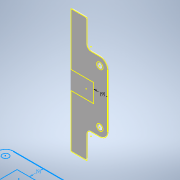
# Autodesk Inventor part: sensor_board
Saved by Autodesk Inventor 2022 (Build 260153000, 153)
## iProperties
Created: 2025-01-11
Part Number: sensor_board
Material: Типовые
Document SubType Name: Modeling
Designer: akap
Density: 1 g/cm^3
Appearance: По умолчанию
Author: akap
Autodesk Inventor part; units mm, degrees
ref_plane "YZ Plane" through (0, 0, 0) normal (1, 0, 0) x (0, 1, 0)
ref_plane "XZ Plane" through (0, 0, 0) normal (0, 1, 0) x (-1, 0, 0)
ref_plane "XY Plane" through (0, 0, 0) normal (0, 0, 1) x (1, 0, 0)
sketch "Эскиз1" plane through (0, 0, 0) normal (0, 0, 1) x (1, 0, 0)
  line L0 (0.35, -40.5) -> (-10.0814, -40.5) projected
  line L1 (0.35, -25.5) -> (0.35, -40.5) projected
  arc A0 (3.05, -22.8) -> (0.35, -25.5) centre (3.05, -25.5) ccw projected
  line L2 (8.75, -22.8) -> (3.05, -22.8) projected
  arc A1 (8.75, -22.8) -> (14.05, -17.5) centre (8.75, -17.5) ccw projected
  line L3 (14.05, 17.5) -> (14.05, -17.5) projected
  arc A2 (14.05, 17.5) -> (8.75, 22.8) centre (8.75, 17.5) ccw projected
  line L4 (3.05, 22.8) -> (8.75, 22.8) projected
  arc A3 (0.35, 25.5) -> (3.05, 22.8) centre (3.05, 25.5) ccw projected
  line L5 (0.35, 40.5) -> (0.35, 25.5) projected
  line L6 (-10.0814, 40.5) -> (0.35, 40.5) projected
  circle A4 centre (8.75, -17.5) radius 2.1 projected
  circle A5 centre (8.75, 17.5) radius 2.1 projected
  line L7 (0.05, -40.2) -> (-10.2488, -40.2)
  line L8 (-10.2488, -40.2) -> (-10.2488, 40.2)
  line L9 (-10.2488, 40.2) -> (0.05, 40.2)
  line L10 (0.05, 40.2) -> (0.05, 25.5)
  arc A6 (0.05, 25.5) -> (3.05, 22.5) centre (3.05, 25.5) ccw
  line L11 (3.05, 22.5) -> (8.75, 22.5)
  arc A7 (13.75, 17.5) -> (8.75, 22.5) centre (8.75, 17.5) ccw
  line L12 (13.75, 17.5) -> (13.75, -17.5)
  arc A8 (8.75, -22.5) -> (13.75, -17.5) centre (8.75, -17.5) ccw
  line L13 (8.75, -22.5) -> (3.05, -22.5)
  arc A9 (3.05, -22.5) -> (0.05, -25.5) centre (3.05, -25.5) ccw
  line L14 (0.05, -25.5) -> (0.05, -40.2)
  circle A10 centre (8.75, -17.5) radius 1.6
  circle A11 centre (8.75, 17.5) radius 1.6
  line L15 (-10.0814, -40.5) -> (-10.0814, -6) projected
  line L16 (-10.0814, 6) -> (-10.0814, 40.5) projected
  line L17 (-10.0814, 6) -> (4.75, 6) projected
  line L18 (4.75, 6) -> (4.75, -6) projected
  line L19 (4.75, -6) -> (-10.0814, -6) projected
  dimension "d7" = 0.3
  dimension "d8" = 3.2
  dimension "d9" = 3.2
  constraints: 16 end point, 8 point on circle, 6 centre point, 2 coincident, 9 other
  measures "d7" distance between parallel lines of L1 L14
  measures "d8" diameter of A10
  measures "d9" diameter of A11
extrude "Выдавливание1" add sketch "Эскиз1" along normal blind 1 contours L15 L19 L18 L17 L16 L9 L10 A6 L11 A7 L12 A8 L13 A9 L14 L7 | L7 L8 L9 L16 L17 L18 L19 L15 | A4 | A5
fillet "Сопряжение1" radius 1 4 edges at (0.05, -40.2, 0.5) (0.05, 40.2, 0.5) (-10.2488, 40.2, 0.5) (-10.2488, -40.2, 0.5)
sketch "Эскиз2" plane through (0, 0, 1) normal (0, 0, 1) x (1, 0, 0)
  circle A0 centre (8.75, -17.5) radius 2.1 projected
  circle A1 centre (8.75, 17.5) radius 2.1 projected
  line L0 (-10.0814, -40.5) -> (-10.0814, -6) projected
  line L1 (0.35, -40.5) -> (-10.0814, -40.5) projected
  line L2 (0.35, -25.5) -> (0.35, -40.5) projected
  arc A2 (3.05, -22.8) -> (0.35, -25.5) centre (3.05, -25.5) ccw projected
  line L3 (8.75, -22.8) -> (3.05, -22.8) projected
  arc A3 (8.75, -22.8) -> (14.05, -17.5) centre (8.75, -17.5) ccw projected
  line L4 (14.05, 17.5) -> (14.05, -17.5) projected
  arc A4 (14.05, 17.5) -> (8.75, 22.8) centre (8.75, 17.5) ccw projected
  line L5 (3.05, 22.8) -> (8.75, 22.8) projected
  arc A5 (0.35, 25.5) -> (3.05, 22.8) centre (3.05, 25.5) ccw projected
  line L6 (0.35, 40.5) -> (0.35, 25.5) projected
  line L7 (-10.0814, 40.5) -> (0.35, 40.5) projected
  line L8 (-10.0814, 6) -> (-10.0814, 40.5) projected
  line L9 (-10.0814, 6) -> (4.75, 6) projected
  line L10 (4.75, 6) -> (4.75, -6) projected
  line L11 (4.75, -6) -> (-10.0814, -6) projected
  line L12 (13.75, -17.5) -> (13.75, 17.5) projected
  point P0 (0, 0)
  dimension "d10" = 9
  measures "d10" distance between parallel lines of L12 L10
